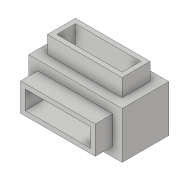
# Autodesk Inventor part: fillet
Saved by Autodesk Inventor 2022 Beta2 (Build 260130000, 130) ContinuousBuild 0
## iProperties
Created: 2018-02-02
Part Number: fillet
Material: Generic
Document SubType Name: Modeling
Designer: jmacmillan
Density: 1 g/cm^3
Appearance: Default
Author: jmacmillan
Autodesk Inventor part; units mm, degrees
ref_plane "YZ Plane" through (0, 0, 0) normal (1, 0, 0) x (0, 1, 0)
ref_plane "XZ Plane" through (0, 0, 0) normal (0, 1, 0) x (-1, 0, 0)
ref_plane "XY Plane" through (0, 0, 0) normal (0, 0, 1) x (1, 0, 0)
sketch "Sketch1" plane through (0, 0, 0) normal (0, 1, 0) x (-1, 0, 0)
  line L0 (200, 100) -> (-200, 100)
  line L1 (-200, 100) -> (-200, -100)
  line L2 (-200, -100) -> (200, -100)
  line L3 (200, -100) -> (200, 100)
  line L4 (0, -140) -> (0, 140) projected
  line L5 (-280, 0) -> (280, 0) projected
  point P0 (0, 0)
  dimension "d0" = 400
  dimension "d1" = 200
  constraints: 8 end point, 2 parallel, 1 horizontal, 1 perpendicular, 2 other
  measures "d0" distance of L2.end L1.end
  measures "d1" distance of L1.end L0.end
extrude "Extrusion1" add sketch "Sketch1" along normal blind 200
sketch "Sketch2" plane through (-200, 0, 100) normal (0, 0, 1) x (1, 0, 0)
  line L0 (0, 0) -> (400, 0) projected
  line L1 (400, 0) -> (400, 200) projected
  line L2 (0, 200) -> (400, 200) projected
  line L3 (0, 0) -> (0, 200) projected
  line L4 (360, 160) -> (360, 40)
  line L5 (360, 40) -> (40, 40)
  line L6 (40, 40) -> (40, 160)
  line L7 (40, 160) -> (360, 160)
  point P0 (200, 0)
  dimension "d4" = 40
  constraints: 8 end point, 3 other
  measures "d4" distance between parallel lines of L2 L7
extrude "Extrusion2" add sketch "Sketch2" along normal blind 75 contours L4 L5 L6 L7
sketch "Sketch3" plane through (-200, 0, 175) normal (0, 0, 1) x (1, 0, 0)
  line L0 (360, 40) -> (360, 160) projected
  line L1 (360, 160) -> (40, 160) projected
  line L2 (40, 160) -> (40, 40) projected
  line L3 (40, 40) -> (360, 40) projected
  line L4 (60, 140) -> (340, 140)
  line L5 (340, 140) -> (340, 60)
  line L6 (340, 60) -> (60, 60)
  line L7 (60, 60) -> (60, 140)
  point P0 (200, 0)
  dimension "d7" = 20
  constraints: 8 end point, 3 other
  measures "d7" distance between parallel lines of L1 L4
extrude "Extrusion3" cut sketch "Sketch3" against normal through all contours L4 L5 L6 L7
sketch "Sketch5" plane through (0, 200, 0) normal (0, 1, 0) x (1, 0, 0)
  line L0 (-200, -100) -> (200, -100) projected
  line L1 (200, -100) -> (200, 100) projected
  line L2 (200, 100) -> (-200, 100) projected
  line L3 (-200, 100) -> (-200, -100) projected
  line L4 (-160, 60) -> (160, 60)
  line L5 (160, 60) -> (160, -60)
  line L6 (160, -60) -> (-160, -60)
  line L7 (-160, -60) -> (-160, 60)
  point P0 (0, 0)
  dimension "d19" = 40
  constraints: 8 end point, 3 other
  measures "d19" distance between parallel lines of L2 L4
extrude "Extrusion4" add sketch "Sketch5" along normal blind 75 contours L4 L5 L6 L7
sketch "Sketch6" plane through (0, 275, 0) normal (0, 1, 0) x (1, 0, 0)
  line L0 (160, 60) -> (-160, 60) projected
  line L1 (-160, 60) -> (-160, -60) projected
  line L2 (-160, -60) -> (160, -60) projected
  line L3 (160, -60) -> (160, 60) projected
  line L4 (-140, 40) -> (140, 40)
  line L5 (140, 40) -> (140, -40)
  line L6 (140, -40) -> (-140, -40)
  line L7 (-140, -40) -> (-140, 40)
  point P0 (0, 0)
  dimension "d22" = 20
  constraints: 8 end point, 3 other
  measures "d22" distance between parallel lines of L0 L4
extrude "Extrusion5" cut sketch "Sketch6" against normal up to surface (135 mm away) contours L4 L5 L6 L7
body "Solid1"
